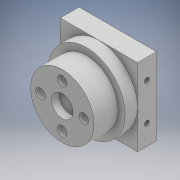
# Autodesk Inventor part: c_axisrot
Saved by Autodesk Inventor 2018 (Build 220112000, 112)
## iProperties
Created: 2018-02-20
Part Number: c_axisrot
Material: Generic
Document SubType Name: Modeling
Designer: Clevo
Density: 1 g/cm^3
Appearance: Default
Author: Clevo
Autodesk Inventor part; units mm, degrees
ref_plane "YZ Plane" through (0, 0, 0) normal (1, 0, 0) x (0, 1, 0)
ref_plane "XZ Plane" through (0, 0, 0) normal (0, 1, 0) x (-1, 0, 0)
ref_plane "XY Plane" through (0, 0, 0) normal (0, 0, 1) x (1, 0, 0)
sketch "Sketch1" plane through (0, 0, 0) normal (0, 1, 0) x (-1, 0, 0)
  circle A0 centre (0, 0) radius 10.25
  dimension "d0" = 20.5
  constraints: 1 centre point, 1 coincident
  measures "d0" diameter of A0
extrude "Extrusion1" add sketch "Sketch1" along normal blind 7.85
sketch "Sketch2" plane through (0, 7.85, 0) normal (0, 1, 0) x (1, 0, 0)
  circle A0 centre (0, 0) radius 12.475
  dimension "d3" = 24.95
  constraints: 1 centre point, 1 coincident
  measures "d3" diameter of A0
extrude "Extrusion2" add sketch "Sketch2" along normal blind 4
sketch "Sketch3" plane through (0, 11.85, 0) normal (0, 1, 0) x (1, 0, 0)
  circle A0 centre (0, 0) radius 12.475 projected
  line L0 (-12.5, -12.5) -> (12.5, -12.5)
  line L1 (12.5, -12.5) -> (12.5, 12.5)
  line L2 (12.5, 12.5) -> (-12.5, 12.5)
  line L3 (-12.5, 12.5) -> (-12.5, -12.5)
  point P0 (-12.5, 0)
  point P1 (0, -12.5)
  dimension "d6" = 25
  dimension "d7" = 25
  constraints: 8 end point, 2 midpoint, 2 parallel, 1 horizontal, 1 horizontal alignment, 1 perpendicular, 1 vertical alignment
  measures "d6" distance of L2.end L0.start
  measures "d7" distance of L1.end L2.end
extrude "Extrusion3" add sketch "Sketch3" along normal blind 6.1 contours A0 | L3 L2 L1 L0
sketch "Sketch4" plane through (12.5, 11.85, 12.5) normal (1, 0, 0) x (0, 0, -1)
  line L0 (0, 0) -> (25, 0) projected
  line L1 (25, 0) -> (25, 6.1) projected
  line L2 (0, 6.1) -> (25, 6.1) projected
  line L3 (0, 0) -> (0, 6.1) projected
  line L4 (24.975, 0) -> (0.025, 0) projected
  line L5 (6.5, 0) -> (18.5, 0)
  line L6 (18.5, 0) -> (18.5, 3)
  line L7 (18.5, 3) -> (6.5, 3)
  line L8 (6.5, 3) -> (6.5, 0)
  point P0 (12.5, -11.85)
  point P1 (12.5, 3)
  point P2 (12.5, 0)
  point P3 (12.5, 0)
  dimension "d10" = 12
  dimension "d11" = 3
  constraints: 8 end point, 3 midpoint, 2 parallel, 2 vertical alignment, 1 horizontal, 1 perpendicular, 1 point on line
  measures "d10" distance of L6.end L7.end
  measures "d11" distance of L7.end L5.start
hole "Hole1" at (12.5, 14.85, 6) at (12.5, 14.85, -6) direction (-1, 0, 0) diameter 1.567 end through all thread size "M2x0.4" class "6H" standard "ANSI Metric M Profile"
sketch "Sketch5" plane through (0, 0, 0) normal (0, -1, 0) x (1, 0, 0)
  circle A0 centre (0, 0) radius 3.5
  dimension "d19" = 7
  constraints: 1 centre point, 1 coincident
  measures "d19" diameter of A0
extrude "Extrusion4" cut sketch "Sketch5" against normal blind 2.5
sketch "Sketch6" plane through (0, 0, 0) normal (0, -1, 0) x (1, 0, 0)
  circle A0 centre (0, 0) radius 7
  line L0 (0, 7) -> (-7, 0)
  line L1 (-7, 0) -> (0, -7)
  line L2 (0, -7) -> (7, 0)
  line L3 (7, 0) -> (0, 7)
  dimension "d22" = 14
  constraints: 8 end point, 2 horizontal alignment, 2 parallel, 2 point on circle, 1 centre point, 1 coincident, 1 perpendicular, 1 vertical alignment
  measures "d22" diameter of A0
hole "Hole2" at (0, 0, 7) at (-7, 0, 0) at (0, 0, -7) at (7, 0, 0) direction (0, 1, 0) diameter 3.1 end through all clearance for "Flat Head Machine Screw" size "M3" standard "Ansi Metric M Profile"
sketch "Sketch7" plane through (0, 17.95, 0) normal (0, 1, 0) x (1, 0, 0)
  circle A0 centre (0, 7) radius 1.55 projected
  circle A1 centre (0, -7) radius 1.55 projected
  circle A2 centre (-7, 0) radius 1.55 projected
  circle A3 centre (7, 0) radius 1.55 projected
  line L0 (-12.5, -12.5) -> (12.5, -12.5) projected
  line L1 (12.5, -12.5) -> (12.5, 12.5) projected
  line L2 (12.5, 12.5) -> (-12.5, 12.5) projected
  line L3 (-12.5, 12.5) -> (-12.5, -12.5) projected
  point P0 (0, 0)
hole "Hole3" at (0, 17.95, 7) at (7, 17.95, 0) at (0, 17.95, -7) at (-7, 17.95, 0) direction (0, -1, 0) diameter 5.7 depth 3.2 tip angle 100
equation "\"d7\" = d6"
body "Solid1"
